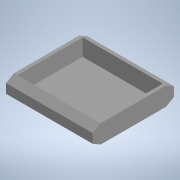
# Autodesk Inventor part: HexBody
Saved by Autodesk Inventor 2020 (Build 240168000, 168)
## iProperties
Created: 2023-12-19
Part Number: HexBody
Material: H TPU
Document SubType Name: Modeling
Designer: smz3rm
Density: 0.941117 g/cm^3
Appearance: Generic(1)
Mass: 209.726 g
Surface Area: 812.475 cm^2
Volume: 222.848 cm^3
BaseThickness: 3.000 mm
TopThickness: 1.000 mm
SideThickness: 6.000 mm
BodyWidth: 160.000 mm
BodyLength: 150.000 mm
BodyHeight: 35.000 mm
DriveMotorHeight: 17.500 mm
WheelWidth: 13.000 mm
WheelGrooveWidth: 3.000 mm
WheelGrooveDia: 22.500 mm
WheelSlotWidth: 16.200 mm
WheelDia: 45.000 mm
WheelPulleyDia: 1.000 mm
Author: smz3rm
Autodesk Inventor part; units mm, degrees
ref_plane "YZ Plane" through (0, 0, 0) normal (1, 0, 0) x (0, 1, 0)
ref_plane "XZ Plane" through (0, 0, 0) normal (0, 1, 0) x (-1, 0, 0)
ref_plane "XY Plane" through (0, 0, 0) normal (0, 0, 1) x (1, 0, 0)
sketch "Sketch1" plane through (0, 0, 0) normal (1, 0, 0) x (0, 1, 0)
  line L0 (-17, 75) -> (17, 75)
  line L1 (17, 75) -> (17, -75)
  line L2 (17, -75) -> (-17, -75)
  line L3 (-17, -75) -> (-17, 75)
  line L4 (-17, 75) -> (17, -75) construction
  line L5 (17, 75) -> (-17, -75) construction
  line L6 (-8.5, 75) -> (8.5, 75)
  line L7 (8.5, 75) -> (17, 60.2776)
  line L8 (17, 60.2776) -> (8.5, 45.5551)
  line L9 (8.5, 45.5551) -> (-8.5, 45.5551)
  line L10 (-8.5, 45.5551) -> (-17, 60.2776)
  line L11 (-17, 60.2776) -> (-8.5, 75)
  line L12 (-23.8, 0) -> (23.8, 0) projected
  line L13 (0, -105) -> (0, 105) projected
  line L14 (8.5, -75) -> (17, -60.2776)
  line L15 (-17, -60.2776) -> (-8.5, -75)
  point P0 (0, 0)
  point P1 (0, 60.2776)
  dimension "d0" = 34
  dimension "d1" = 150
  constraints: 28 end point, 4 point on line, 4 symmetric about line, 2 midpoint, 2 parallel, 1 horizontal, 1 perpendicular, 13 other
  measures "d0" distance of L1.end L2.end
  measures "d1" distance of L0.end L1.end
extrude "Extrusion1" add sketch "Sketch1" along normal mid plane 160 contours L0 L13 L9 L10 L11 | L10 L9 L13 L12 L3 | L0 L7 L8 L9 L13 | L12 L13 L2 L15 L3 | L9 L8 L1 L12 L13 | L12 L1 L14 L2 L13
sketch "Sketch2" plane through (-80, 17, 60.2776) normal (0, 1, 0) x (1, 0, 0)
  line L0 (0, 0) -> (160, 0) projected
  line L1 (160, 120.5551) -> (160, 0) projected
  line L2 (160, 120.5551) -> (0, 120.5551) projected
  line L3 (0, 0) -> (0, 120.5551) projected
  line L4 (0, 0) -> (160, 0) projected
  line L5 (154, 120.5551) -> (6, 120.5551)
  line L6 (6, 120.5551) -> (6, 0)
  line L7 (6, 0) -> (154, 0)
  line L8 (154, 0) -> (154, 120.5551)
  line L9 (154, 120.5551) -> (6, 0) construction
  line L10 (6, 120.5551) -> (154, 0) construction
  point P0 (80, 60.2776)
  point P1 (6, 120.5551)
  point P2 (6, 0)
  dimension "d4" = 6
  constraints: 12 end point, 2 midpoint, 2 parallel, 1 horizontal, 1 perpendicular, 1 point on line
  measures "d4" distance between parallel lines of L3 L6
extrude "Extrusion2" cut sketch "Sketch2" against normal blind 31 contours L6 L2 L8 L0
equation "\"d0\" = BodyHeight - TopThickness"
equation "\"d1\" = BodyLength"
equation "\"d2\" = BodyWidth"
equation "\"d4\" = SideThickness"
equation "\"d5\" = -TopThickness + BodyHeight - BaseThickness"
equation "\"BaseThickness\" = 3"
equation "\"TopThickness\" = 1"
equation "\"SideThickness\" = 6"
equation "\"BodyWidth\" = 160"
equation "\"BodyLength\" = 150"
equation "\"BodyHeight\" = 35"
equation "\"DriveMotorHeight\" = 0.5 * BodyHeight"
equation "\"WheelWidth\" = 13"
equation "\"WheelGrooveWidth\" = 3"
equation "\"WheelGrooveDia\" = 0.5 * WheelDia"
equation "\"WheelPulleyDia\" = 1"
equation "\"WheelDia\" = 45"
body "Solid1"
